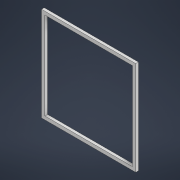
# Autodesk Inventor part: Shoulder_Cube_TestFit_V1
Saved by Autodesk Inventor 2022 (Build 260153000, 153)
## iProperties
Created: 2023-05-16
Part Number: Shoulder_Cube_TestFit_V1
Material: Generic
Document SubType Name: Modeling
Designer: Karl Spiteri
Density: 1 g/cm^3
Appearance: Default
Author: Karl Spiteri
Autodesk Inventor part; units mm, degrees
ref_plane "YZ Plane" through (0, 0, 0) normal (1, 0, 0) x (0, 1, 0)
ref_plane "XZ Plane" through (0, 0, 0) normal (0, 1, 0) x (-1, 0, 0)
ref_plane "XY Plane" through (0, 0, 0) normal (0, 0, 1) x (1, 0, 0)
sketch "Sketch1" plane through (0, 0, 0) normal (0, 0, 1) x (1, 0, 0)
  line L0 (0, 0) -> (-70, 0)
  line L1 (-70, 0) -> (-70, 70)
  line L2 (-70, 70) -> (0, 70)
  line L3 (0, 70) -> (0, 0)
  line L4 (-2.5, 2.5) -> (-67.5, 2.5)
  line L5 (-67.5, 2.5) -> (-67.5, 67.5)
  line L6 (-67.5, 67.5) -> (-2.5, 67.5)
  line L7 (-2.5, 67.5) -> (-2.5, 2.5)
  dimension "d0" = 70
  dimension "d1" = 70
  dimension "d6" = 65
  dimension "d7" = 65
  constraints: 16 end point, 4 parallel, 2 horizontal, 2 perpendicular
  measures "d0" distance of L1.end L2.end
  measures "d1" distance of L0.end L1.end
  measures "d6" distance of L5.end L6.end
  measures "d7" distance of L4.end L5.end
extrude "Extrusion2" add sketch "Sketch1" along normal blind 2
body "Solid2"
